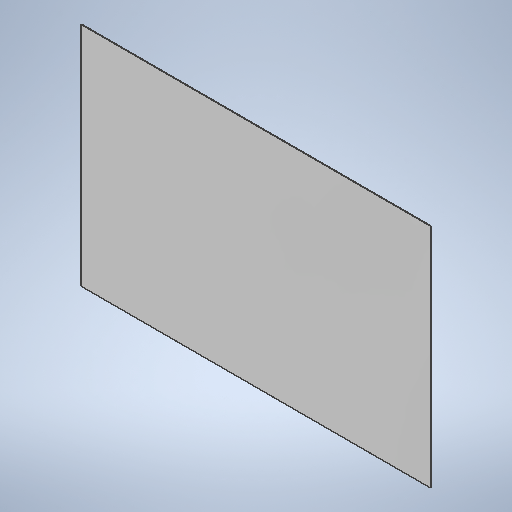
# Autodesk Inventor part: PLANCHA DE CRISTAL DE ESPEJO 3300x2140 mm
Saved by Autodesk Inventor 2025 (Build 290162000, 162)
## iProperties
Created: 2026-02-16
Part Number: PLANCHA DE CRISTAL DE ESPEJO 3300x2140 mm
Material: Cristal
Document SubType Name: Modeling
Designer: Frank
Density: 2.18 g/cm^3
Appearance: De espejo
Author: Frank
Autodesk Inventor part; units mm, degrees
ref_plane "YZ Plane" through (0, 0, 0) normal (1, 0, 0) x (0, 1, 0)
ref_plane "XZ Plane" through (0, 0, 0) normal (0, 1, 0) x (-1, 0, 0)
ref_plane "XY Plane" through (0, 0, 0) normal (0, 0, 1) x (1, 0, 0)
sketch "Boceto1" plane through (0, 0, 0) normal (0, 0, 1) x (1, 0, 0)
  line L0 (-1827.3364, 1385.9229) -> (1472.6636, 1385.9229)
  line L1 (1472.6636, 1385.9229) -> (1472.6636, -754.0771)
  line L2 (1472.6636, -754.0771) -> (-1827.3364, -754.0771)
  line L3 (-1827.3364, -754.0771) -> (-1827.3364, 1385.9229)
  point P0 (0, 0)
  dimension "d2" = 3300
  dimension "d3" = 2140
  constraints: 8 end point, 2 parallel, 1 horizontal, 1 perpendicular
  measures "d2" distance of L0.start L0.end
  measures "d3" distance of L2.end L0.start
extrude "Extrusión1" add sketch "Boceto1" along normal blind 5
